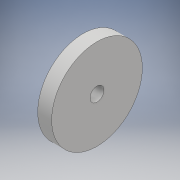
# Autodesk Inventor part: rosquilla
Saved by Autodesk Inventor 2018 (Build 220112000, 112)
## iProperties
Created: 2020-03-10
Part Number: rosquilla
Material: Genérico
Document SubType Name: Modeling
Designer: sala.ceri
Density: 1 g/cm^3
Appearance: Valor por defecto
Author: sala.ceri
Autodesk Inventor part; units mm, degrees
ref_plane "YZ Plane" through (0, 0, 0) normal (1, 0, 0) x (0, 1, 0)
ref_plane "XZ Plane" through (0, 0, 0) normal (0, 1, 0) x (-1, 0, 0)
ref_plane "XY Plane" through (0, 0, 0) normal (0, 0, 1) x (1, 0, 0)
sketch "Boceto1" plane through (0, 0, 0) normal (1, 0, 0) x (0, 1, 0)
  circle A0 centre (0, 0) radius 9.75
  circle A1 centre (0, 0) radius 1.5
  dimension "d2" = 3
  constraints: 2 centre point, 1 coincident
extrude "Extrusión1" add sketch "Boceto1" along normal blind 3
